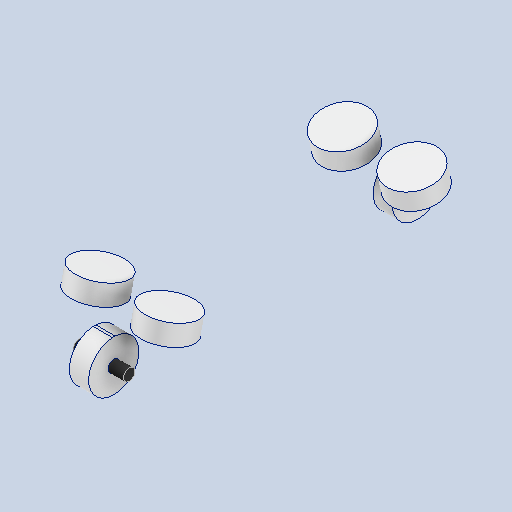
# Autodesk Inventor part: belt_liner_v2_B_unit-2
Saved by Autodesk Inventor 2025.2 (Build 292293000, 293)
## iProperties
Created: 2025-01-06
Part Number: belt_liner_v2_B_unit-2
Material: アルミニウム 6061
Document SubType Name: Modeling
Designer: haruy
Density: 2.7 g/cm^3
Appearance: アルミニウム - フラット
Author: haruy
Autodesk Inventor part; units mm, degrees
ref_plane "YZ Plane" through (0, 0, 0) normal (1, 0, 0) x (0, 1, 0)
ref_plane "XZ Plane" through (0, 0, 0) normal (0, 1, 0) x (-1, 0, 0)
ref_plane "XY Plane" through (0, 0, 0) normal (0, 0, 1) x (1, 0, 0)
derived "base_weel-v2-Sketch-Base.ipt"
ref_plane "作業平面1" through (0, 0, 0) normal (1, 0, 0) x (0, 1, 0)
ref_plane "作業平面2" through (-9, 0, 0) normal (1, 0, 0) x (0, 1, 0)
sketch "スケッチ1" plane through (0, 0, 0) normal (1, 0, 0) x (0, 1, 0)
  line L0 (-315, 315) -> (315, 315) projected
  line L1 (315, 315) -> (315, -315) projected
  line L2 (315, -315) -> (-315, -315) projected
  line L3 (-315, -315) -> (-315, 315) projected
  line L4 (-315, 315) -> (315, -315) construction
  line L5 (315, 315) -> (-315, -315) construction
  line L6 (-315, 210) -> (-300, 210) projected
  line L7 (-300, 210) -> (-300, -210) projected
  line L8 (-300, -210) -> (-315, -210) projected
  line L9 (-315, -210) -> (-315, 210) projected
  line L10 (242, 315) -> (-242, 315) projected
  line L11 (-242, 315) -> (-242, 295) projected
  line L12 (-242, 295) -> (242, 295) projected
  line L13 (242, 295) -> (242, 315) projected
  line L14 (-300, 210) -> (-300, 315) projected
  line L15 (0, 0) -> (-956.5973, 0) projected
  circle A0 centre (0, 0) radius 400 projected
  line L16 (-330, 25) -> (-380, 25) projected
  line L17 (-380, 25) -> (-380, -25) projected
  line L18 (-380, -25) -> (-330, -25) projected
  line L19 (-330, -25) -> (-330, 25) projected
  line L20 (0, 0) -> (0, -630.9179) projected
  line L21 (-315, 40) -> (-395, 40) projected
  line L22 (-395, 40) -> (-395, 30) projected
  line L23 (-395, 30) -> (-315, 30) projected
  line L24 (-315, 30) -> (-315, 40) projected
  line L25 (-395, 30) -> (-385, 30) projected
  line L26 (-385, 30) -> (-385, 0) projected
  line L27 (-385, 0) -> (-395, 0) projected
  line L28 (-395, 0) -> (-395, 30) projected
  line L29 (300, 210) -> (315, 210) projected
  line L30 (315, 210) -> (315, -210) projected
  line L31 (315, -210) -> (300, -210) projected
  line L32 (300, -210) -> (300, 210) projected
  line L33 (-222.2183, -315) -> (242, -315) projected
  line L34 (242, -315) -> (242, -295) projected
  line L35 (242, -295) -> (-242, -295) projected
  line L36 (315, 315) -> (0, 0) projected
  line L37 (315, 125) -> (315, 145) projected
  circle A1 centre (512, 0) radius 122.5 projected
  circle A2 centre (179.6905, 0) radius 600 projected
  circle A3 centre (541.6815, 0) radius 200 projected
  circle A4 centre (0, 0) radius 10 projected
  arc A5 (0, 150) -> (0, -150) centre (0, 0) ccw projected
  arc A6 (0, 140) -> (0, -140) centre (0, 0) ccw projected
  line L38 (-146.3272, 32.9904) -> (-136.572, 30.791) projected
  line L39 (-137.5812, 37.6817) -> (-140.4404, 25) projected
  line L40 (-140.4404, 25) -> (-145.318, 26.0997) projected
  line L41 (-145.318, 26.0997) -> (-142.4588, 38.7814) projected
  line L42 (-142.4588, 38.7814) -> (-137.5812, 37.6817) projected
  arc A7 (-29.1302, 142.0438) -> (-29.1302, -142.0438) centre (0, 0) ccw projected
  circle A8 centre (-151.4904, 39.2799) radius 6.5 projected
  circle A9 centre (-129.0401, 34.2184) radius 6.5 projected
  circle A10 centre (-129.0401, 34.2184) radius 1.5 projected
  circle A11 centre (-151.4904, 39.2799) radius 1.5 projected
  line L43 (-104.1709, 22.5) -> (-174.1362, 22.5) projected
  line L44 (-174.1362, 22.5) -> (-174.1362, 7.5) projected
  line L45 (-174.1362, 7.5) -> (-104.1709, 7.5) projected
  line L46 (-104.1709, 7.5) -> (-104.1709, 22.5) projected
  circle A12 centre (-129.0401, -34.2184) radius 6.5 projected
  circle A13 centre (-129.0401, -34.2184) radius 1.5 projected
  line L47 (-142.4588, -38.7814) -> (-137.5812, -37.6817) projected
  line L48 (-145.318, -26.0997) -> (-142.4588, -38.7814) projected
  line L49 (-137.5812, -37.6817) -> (-140.4404, -25) projected
  line L50 (-140.4404, -25) -> (-145.318, -26.0997) projected
  circle A14 centre (-151.4904, -39.2799) radius 6.5 projected
  circle A15 centre (-151.4904, -39.2799) radius 1.5 projected
  line L51 (-146.3272, -32.9904) -> (-136.572, -30.791) projected
  line L52 (-104.1709, -22.5) -> (-174.1362, -22.5) projected
  line L53 (-174.1362, -7.5) -> (-104.1709, -7.5) projected
  line L54 (-104.1709, -7.5) -> (-104.1709, -22.5) projected
  line L55 (-174.1362, -22.5) -> (-174.1362, -7.5) projected
  line L56 (-151.4904, 39.2799) -> (-129.0401, 34.2184) construction
  line L57 (-129.0401, 34.2184) -> (-129.59, 31.7796) construction
  line L58 (-129.59, 31.7796) -> (-152.0402, 36.8412) construction
  line L59 (-152.0402, 36.8412) -> (-151.4904, 39.2799) construction
  line L60 (-129.0401, 34.2184) -> (-151.4904, 39.2799) construction
  line L61 (-151.4904, 39.2799) -> (-150.9405, 41.7187) construction
  line L62 (-150.9405, 41.7187) -> (-128.4903, 36.6572) construction
  line L63 (-128.4903, 36.6572) -> (-129.0401, 34.2184) construction
  line L64 (-128.4903, 36.6572) -> (-129.59, 31.7796) construction
  line L65 (-129.59, 31.7796) -> (-117.8838, 29.1404) construction
  line L66 (-117.8838, 29.1404) -> (-116.7841, 34.0179) construction
  line L67 (-116.7841, 34.0179) -> (-128.4903, 36.6572) construction
  line L68 (-150.9405, 41.7187) -> (-152.0402, 36.8412) construction
  line L69 (-152.0402, 36.8412) -> (-163.7464, 39.4804) construction
  line L70 (-163.7464, 39.4804) -> (-162.6467, 44.358) construction
  line L71 (-162.6467, 44.358) -> (-150.9405, 41.7187) construction
  line L72 (-155.2683, 45.2572) -> (-128.9412, 39.3216) projected
  line L73 (-128.9412, 39.3216) -> (-132.2403, 24.6889) projected
  line L74 (-132.2403, 24.6889) -> (-158.5673, 30.6245) projected
  line L75 (-158.5673, 30.6245) -> (-155.2683, 45.2572) projected
  line L76 (-128.9412, -39.3216) -> (-132.2403, -24.6889) projected
  line L77 (-155.2683, -45.2572) -> (-128.9412, -39.3216) projected
  line L78 (-132.2403, -24.6889) -> (-158.5673, -30.6245) projected
  line L79 (-158.5673, -30.6245) -> (-155.2683, -45.2572) projected
  arc A16 (-132.2403, 24.6889) -> (-132.2403, -24.6889) centre (0, 0) ccw projected
  arc A17 (-158.5673, 30.6245) -> (-158.5673, -30.6245) centre (0, 0) ccw projected
  circle A18 centre (-152.5, 15) radius 1.25 projected
  line L80 (-145, 0) -> (-145, 74.7382) projected
  circle A19 centre (-137.5, 15) radius 1.25 projected
  circle A20 centre (-137.5, -15) radius 1.25 projected
  circle A21 centre (-152.5, -15) radius 1.25 projected
  line L81 (0, 0) -> (0, 140) projected
  line L82 (0, 0) -> (-47.8828, 131.557) projected
  line L83 (0, 140) -> (0, 150) projected
  line L84 (-137.5846, 25.8938) -> (-134.2855, 40.5265) projected
  line L85 (-137.5846, -25.8938) -> (-134.2855, -40.5265) projected
  circle A22 centre (0, 0) radius 20 projected
  line L86 (300, 70) -> (-300, 70) projected
  line L87 (-300, 70) -> (-300, 50) projected
  line L88 (-300, 50) -> (300, 50) projected
  line L89 (300, 50) -> (300, 70) projected
  line L90 (-40, 295) -> (-60, 295) projected
  line L91 (-60, 295) -> (-60, 70) projected
  line L92 (-60, 70) -> (-40, 70) projected
  line L93 (-40, 70) -> (-40, 295) projected
  line L94 (-60, -295) -> (-60, -70) projected
  line L95 (-40, -70) -> (-40, -295) projected
  line L96 (300, -70) -> (-300, -70) projected
  line L97 (-300, -50) -> (300, -50) projected
  line L98 (-40, 70) -> (-40, -70) projected
  line L99 (40, 70) -> (40, -70) projected
  circle A23 centre (20, 60) radius 1.5 projected
  circle A24 centre (-20, 60) radius 1.5 projected
  circle A25 centre (-20, -60) radius 1.5 projected
  circle A26 centre (20, -60) radius 1.5 projected
  circle A27 centre (-50, 125) radius 1.5 projected
  circle A28 centre (-50, 125) radius 5 projected
  circle A29 centre (-120, 60) radius 5 projected
  circle A30 centre (-120, 60) radius 1.5 projected
  line L100 (-40, 134.1641) -> (-45.5009, 122.8186) projected
  line L101 (-53.0865, 121.0664) -> (-60, 126.4911) projected
  line L102 (-130.767, 50) -> (-118.047, 55.3972) projected
  line L103 (-121.2436, 70) -> (-115.9982, 62.9976) projected
  line L104 (-40, -134.1641) -> (-45.5009, -122.8186) projected
  circle A31 centre (-50, -125) radius 5 projected
  circle A32 centre (-50, -125) radius 1.5 projected
  line L105 (-53.0865, -121.0664) -> (-60, -126.4911) projected
  line L106 (-121.2436, -70) -> (-115.9982, -62.9976) projected
  circle A33 centre (-120, -60) radius 5 projected
  circle A34 centre (-120, -60) radius 1.5 projected
  line L107 (-130.767, -50) -> (-118.047, -55.3972) projected
  line L108 (-242, -295) -> (-242, -315) projected
  line L109 (242, 315) -> (222, 315) projected
  line L110 (222, 315) -> (222, 295) projected
  line L111 (222, 295) -> (242, 295) projected
  line L112 (242, 295) -> (242, 315) projected
  line L113 (242, -315) -> (222, -315) projected
  line L114 (222, -315) -> (222, -295) projected
  line L115 (222, -295) -> (242, -295) projected
  line L116 (242, -295) -> (242, -315) projected
  line L117 (212, 295) -> (300, 207) projected
  line L118 (300, 207) -> (289.3934, 196.3934) projected
  line L119 (289.3934, 196.3934) -> (201.3934, 284.3934) projected
  line L120 (201.3934, 284.3934) -> (212, 295) projected
  line L121 (212, 295) -> (212, 315) projected
  line L122 (213.5485, 293.4515) -> (202.9419, 282.8449) projected
  line L123 (205.7703, 280.0165) -> (280.0165, 205.7703) projected
  line L124 (280.0165, 205.7703) -> (239.0043, 164.7581) projected
  line L125 (239.0043, 164.7581) -> (164.7581, 239.0043) projected
  line L126 (164.7581, 239.0043) -> (205.7703, 280.0165) projected
  line L127 (298.4013, 208.5987) -> (287.7947, 197.9921) projected
  line L128 (111.018, 292.7444) -> (296.9871, 106.7753) projected
  line L129 (296.9871, 106.7753) -> (286.3805, 96.1687) projected
  line L130 (286.3805, 96.1687) -> (100.4114, 282.1378) projected
  line L131 (100.4114, 282.1378) -> (111.018, 292.7444) projected
  line L132 (221.6802, 285.3198) -> (211.0736, 274.7132) projected
  line L133 (285.3198, 221.6802) -> (274.7132, 211.0736) projected
  circle A35 centre (211.7807, 284.6127) radius 1.5 projected
  circle A36 centre (222.3873, 274.0061) radius 1.5 projected
  circle A37 centre (289.5624, 206.831) radius 1.5 projected
  circle A38 centre (275.4203, 220.9731) radius 1.5 projected
  circle A39 centre (112.7858, 280.3701) radius 1.5 projected
  circle A40 centre (119.8568, 273.299) radius 1.5 projected
  circle A41 centre (284.6127, 108.5431) radius 1.5 projected
  circle A42 centre (277.5416, 115.6142) radius 1.5 projected
  line L134 (201.3934, 284.3934) -> (190.7868, 295) projected
  circle A43 centre (202, 305) radius 1.5 projected
  circle A44 centre (192, 305) radius 1.5 projected
  line L135 (187, 315) -> (187, 295) projected
  line L136 (111.018, 292.7444) -> (108.7624, 295) projected
  line L137 (108.7624, 295) -> (108.7624, 315) projected
  line L138 (100.4114, 282.1378) -> (87.5492, 295) projected
  circle A45 centre (98.7624, 305) radius 1.5 projected
  circle A46 centre (88.7624, 305) radius 1.5 projected
  line L139 (83.7624, 315) -> (83.7624, 295) projected
  circle A47 centre (307.5, 197) radius 1.5 projected
  circle A48 centre (307.5, 187) radius 1.5 projected
  line L140 (289.3934, 196.3934) -> (300, 185.7868) projected
  line L141 (300, 207) -> (315, 207) projected
  line L142 (315, 182) -> (300, 182) projected
  line L143 (296.9871, 106.7753) -> (300, 103.7624) projected
  line L144 (286.3805, 96.1687) -> (300, 82.5492) projected
  line L145 (300, 103.7624) -> (315, 103.7624) projected
  circle A49 centre (307.5, 93.7624) radius 1.5 projected
  circle A50 centre (307.5, 83.7624) radius 1.5 projected
  line L146 (300, 78.7624) -> (315, 78.7624) projected
  line L147 (-212, 295) -> (-212, 315) projected
  circle A51 centre (-202, 305) radius 1.5 projected
  circle A52 centre (-192, 305) radius 1.5 projected
  line L148 (-187, 315) -> (-187, 295) projected
  line L149 (-108.7624, 295) -> (-108.7624, 315) projected
  circle A53 centre (-98.7624, 305) radius 1.5 projected
  circle A54 centre (-88.7624, 305) radius 1.5 projected
  line L150 (-83.7624, 315) -> (-83.7624, 295) projected
  line L151 (-100.4114, 282.1378) -> (-87.5492, 295) projected
  line L152 (-111.018, 292.7444) -> (-108.7624, 295) projected
  line L153 (-111.018, 292.7444) -> (-296.9871, 106.7753) projected
  line L154 (-100.4114, 282.1378) -> (-111.018, 292.7444) projected
  line L155 (-286.3805, 96.1687) -> (-100.4114, 282.1378) projected
  circle A55 centre (-112.7858, 280.3701) radius 1.5 projected
  circle A56 centre (-119.8568, 273.299) radius 1.5 projected
  line L156 (-296.9871, 106.7753) -> (-286.3805, 96.1687) projected
  line L157 (-296.9871, 106.7753) -> (-300, 103.7624) projected
  line L158 (-286.3805, 96.1687) -> (-300, 82.5492) projected
  line L159 (-300, 78.7624) -> (-315, 78.7624) projected
  line L160 (-300, 103.7624) -> (-315, 103.7624) projected
  circle A57 centre (-307.5, 93.7624) radius 1.5 projected
  circle A58 centre (-307.5, 83.7624) radius 1.5 projected
  line L161 (-280.0165, 205.7703) -> (-239.0043, 164.7581) projected
  line L162 (-164.7581, 239.0043) -> (-205.7703, 280.0165) projected
  line L163 (-289.3934, 196.3934) -> (-201.3934, 284.3934) projected
  line L164 (-201.3934, 284.3934) -> (-190.7868, 295) projected
  line L165 (-212, 295) -> (-300, 207) projected
  line L166 (-213.5485, 293.4515) -> (-202.9419, 282.8449) projected
  line L167 (-221.6802, 285.3198) -> (-211.0736, 274.7132) projected
  circle A59 centre (-275.4203, 220.9731) radius 1.5 projected
  circle A60 centre (-289.5624, 206.831) radius 1.5 projected
  line L168 (-298.4013, 208.5987) -> (-287.7947, 197.9921) projected
  line L169 (-289.3934, 196.3934) -> (-300, 185.7868) projected
  line L170 (-300, 207) -> (-315, 207) projected
  circle A61 centre (-307.5, 197) radius 1.5 projected
  circle A62 centre (-307.5, 187) radius 1.5 projected
  line L171 (-315, 182) -> (-300, 182) projected
  circle A63 centre (-275.4203, 220.9731) radius 1.5 projected
  circle A64 centre (-289.5624, 206.831) radius 1.5 projected
  circle A65 centre (-211.7807, 284.6127) radius 1.5 projected
  circle A66 centre (-222.3873, 274.0061) radius 1.5 projected
  circle A67 centre (-307.5, -93.7624) radius 1.5 projected
  circle A68 centre (-307.5, -83.7624) radius 1.5 projected
  circle A69 centre (-307.5, -187) radius 1.5 projected
  circle A70 centre (-307.5, -197) radius 1.5 projected
  line L172 (-111.018, -292.7444) -> (-296.9871, -106.7753) projected
  line L173 (-286.3805, -96.1687) -> (-100.4114, -282.1378) projected
  line L174 (-296.9871, -106.7753) -> (-286.3805, -96.1687) projected
  line L175 (-212, -295) -> (-300, -207) projected
  line L176 (-289.3934, -196.3934) -> (-201.3934, -284.3934) projected
  circle A71 centre (-289.5624, -206.831) radius 1.5 projected
  circle A72 centre (-275.4203, -220.9731) radius 1.5 projected
  line L177 (-298.4013, -208.5987) -> (-287.7947, -197.9921) projected
  circle A73 centre (-222.3873, -274.0061) radius 1.5 projected
  line L178 (-221.6802, -285.3198) -> (-211.0736, -274.7132) projected
  line L179 (-213.5485, -293.4515) -> (-202.9419, -282.8449) projected
  circle A74 centre (-211.7807, -284.6127) radius 1.5 projected
  circle A75 centre (-119.8568, -273.299) radius 1.5 projected
  circle A76 centre (-112.7858, -280.3701) radius 1.5 projected
  line L180 (-100.4114, -282.1378) -> (-111.018, -292.7444) projected
  circle A77 centre (-202, -305) radius 1.5 projected
  circle A78 centre (-192, -305) radius 1.5 projected
  circle A79 centre (-98.7624, -305) radius 1.5 projected
  circle A80 centre (-88.7624, -305) radius 1.5 projected
  circle A81 centre (98.7624, -305) radius 1.5 projected
  circle A82 centre (88.7624, -305) radius 1.5 projected
  line L181 (286.3805, -96.1687) -> (100.4114, -282.1378) projected
  line L182 (100.4114, -282.1378) -> (111.018, -292.7444) projected
  line L183 (111.018, -292.7444) -> (296.9871, -106.7753) projected
  circle A83 centre (112.7858, -280.3701) radius 1.5 projected
  circle A84 centre (119.8568, -273.299) radius 1.5 projected
  circle A85 centre (192, -305) radius 1.5 projected
  circle A86 centre (202, -305) radius 1.5 projected
  line L184 (289.3934, -196.3934) -> (201.3934, -284.3934) projected
  line L185 (213.5485, -293.4515) -> (202.9419, -282.8449) projected
  line L186 (212, -295) -> (300, -207) projected
  circle A87 centre (211.7807, -284.6127) radius 1.5 projected
  circle A88 centre (222.3873, -274.0061) radius 1.5 projected
  circle A89 centre (275.4203, -220.9731) radius 1.5 projected
  circle A90 centre (289.5624, -206.831) radius 1.5 projected
  line L187 (298.4013, -208.5987) -> (287.7947, -197.9921) projected
  circle A91 centre (307.5, -197) radius 1.5 projected
  circle A92 centre (307.5, -187) radius 1.5 projected
  line L188 (296.9871, -106.7753) -> (286.3805, -96.1687) projected
  circle A93 centre (284.6127, -108.5431) radius 1.5 projected
  circle A94 centre (277.5416, -115.6142) radius 1.5 projected
  circle A95 centre (307.5, -93.7624) radius 1.5 projected
  circle A96 centre (307.5, -83.7624) radius 1.5 projected
  circle A97 centre (-284.6127, 108.5431) radius 1.5 projected
  circle A98 centre (-277.5416, 115.6142) radius 1.5 projected
  circle A99 centre (-284.6127, -108.5431) radius 1.5 projected
  circle A100 centre (-277.5416, -115.6142) radius 1.5 projected
  line L189 (242, 295) -> (222, 295) projected
  line L190 (222, 295) -> (222, 243) projected
  line L191 (222, 243) -> (242, 243) projected
  line L192 (242, 243) -> (242, 295) projected
  point P0 (-141.4496, 31.8907)
  point P1 (-129.0401, 34.2184)
  point P2 (-139.0108, 31.3408)
  point P3 (-143.8884, 32.4405)
  point P4 (-143.8884, -32.4405)
  point P5 (-139.0108, -31.3408)
  point P6 (-145, 38.9265)
  point P7 (-145, 39.6334)
  point P8 (-150, 0)
  point P9 (-242, 305)
  constraints: 1 other
revolve "回転1" add sketch "スケッチ1" angle 360 about axis through (0, -146.3272, 32.9904) along (0, 0.9755144, -0.2199357) contours A7 L38 L41 L42 | L42 L39 L38 A7
revolve "回転2" add sketch "スケッチ1" angle 360 about axis through (0, -146.3272, -32.9904) along (0, 0.9755144, 0.2199357) separate body contours L48 L78 A7 L51 | A7 L78 L49 L51 | L50 L49 L78 A7 | A7 L78 L48 L50
extrude "押し出し1" add sketch "スケッチ1" along normal mid plane 5 from surface at -9 separate body contours L72 A8 | A8 L80 L75 L72 | A14 L77 L79 | A14 L77 | L79 A14 | A8 L75 picked at (-150.697, -43.028)
extrude "押し出し2" add sketch "スケッチ1" along normal mid plane 13 from surface at -9 separate body contours A11 | A15
mirror "ミラー1" about plane through (-9, 0, 0) normal (1, 0, 0) bodies 1 2
